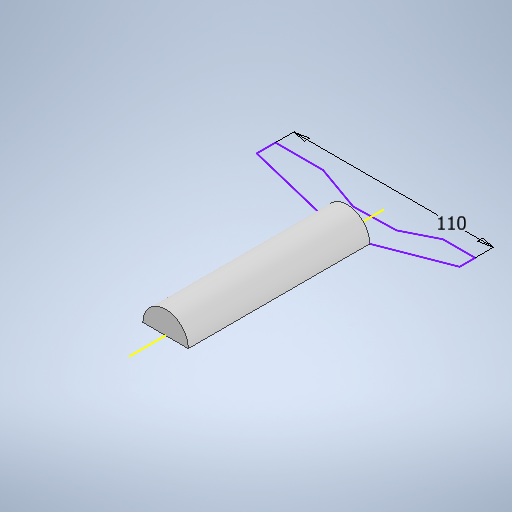
# Autodesk Inventor part: prop
Saved by Autodesk Inventor 2025.2 (Build 292293000, 293)
## iProperties
Created: 2025-03-24
Part Number: prop
Material: Všeobecné
Document SubType Name: Modeling
Designer: hepma_axt67em
Density: 1 g/cm^3
Appearance: Výchozí
Author: hepma_axt67em
Autodesk Inventor part; units mm, degrees
ref_plane "YZ Plane" through (0, 0, 0) normal (1, 0, 0) x (0, 1, 0)
ref_plane "XZ Plane" through (0, 0, 0) normal (0, 1, 0) x (-1, 0, 0)
ref_plane "XY Plane" through (0, 0, 0) normal (0, 0, 1) x (1, 0, 0)
sketch "Náčrt1" plane through (0, 0, 0) normal (0, 0, 1) x (1, 0, 0)
  line L0 (0, 15) -> (0, -2.5) projected
  arc A0 (12.5, 0) -> (-12.5, 0) centre (0, 0) ccw
  line L1 (-17.5, 0) -> (17.5, 0) projected
  line L2 (12.5, 0) -> (-12.5, 0)
  dimension "d0" = 12.5
  constraints: 2 end point, 2 point on circle, 1 centre point, 1 coincident, 1 collinear
  measures "d0" radius of A0
extrude "Vysunutí1" add sketch "Náčrt1" along normal mid plane 100
sketch "Náčrt2" plane through (0, 0, 0) normal (0, 1, 0) x (-1, 0, 0)
  line L0 (-12.5, -50) -> (12.5, -50) projected
  line L1 (0, -70) -> (0, 70) projected
  line L2 (12.5, -50) -> (61.7815, -62.0121)
  line L3 (61.7815, -62.0121) -> (61.7815, -72.33)
  line L4 (61.7815, -72.33) -> (35.5901, -72.33)
  line L5 (35.5901, -72.33) -> (9.8325, -63.1998)
  line L6 (9.8325, -63.1998) -> (-13.4756, -63.7936)
  line L7 (-13.4756, -63.7936) -> (-30.4741, -72.33)
  line L8 (-30.4741, -72.33) -> (-48.2185, -72.33)
  line L9 (-48.2185, -72.33) -> (-48.2185, -63.7936)
  line L10 (-48.2185, -63.7936) -> (-12.5, -50)
  line L11 (12.5, -50) -> (-12.5, -50)
  point P0 (0, 0)
  dimension "d4" = 110
  constraints: 20 end point, 3 perpendicular, 1 point on line, 1 vertical
  measures "d4" distance between parallel lines of L9 L3
